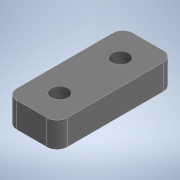
# Autodesk Inventor part: BeltClip
Saved by Autodesk Inventor 2022 (Build 260153000, 153)
## iProperties
Created: 2021-06-25
Part Number: BeltClip
Material: Generic
Document SubType Name: Modeling
Designer: BBL
Density: 1 g/cm^3
Appearance: Gray
Author: BBL
Autodesk Inventor part; units mm, degrees
ref_plane "YZ Plane" through (0, 0, 0) normal (1, 0, 0) x (0, 1, 0)
ref_plane "XZ Plane" through (0, 0, 0) normal (0, 1, 0) x (-1, 0, 0)
ref_plane "XY Plane" through (0, 0, 0) normal (0, 0, 1) x (1, 0, 0)
sketch "Sketch1" plane through (0, 0, 0) normal (0, 1, 0) x (-1, 0, 0)
  circle A0 centre (0, 0) radius 1.65
  circle A1 centre (0, -12) radius 1.65
  line L0 (-5, 5.5) -> (5, 5.5)
  line L1 (5, 5.5) -> (5, -17.5)
  line L2 (5, -17.5) -> (-5, -17.5)
  line L3 (-5, -17.5) -> (-5, 5.5)
  dimension "d0" = 3.3
  dimension "d1" = 3.3
  dimension "d2" = 12
  dimension "d3" = 0
  dimension "d4" = 10
  dimension "d5" = 5
  dimension "d6" = 5.5
  dimension "d7" = 5.5
  constraints: 8 end point, 2 centre point, 2 parallel, 1 coincident, 1 horizontal, 1 perpendicular
  measures "d0" diameter of A0
  measures "d1" diameter of A1
  measures "d2" distance of A1.centre point (0, 0)
  measures "d3" horizontal distance of point (0, 0) A1.centre
  measures "d4" distance of L0.start L0.end
  measures "d5" distance from line of point (0, 0) L3
  measures "d6" distance from line of point (0, 0) L0
  measures "d7" distance from line of L2 A1.centre
extrude "Extrusion1" add sketch "Sketch1" along normal blind 5
fillet "Fillet1" radius 2 4 edges at (5, 2.5, 5.5) (-5, 2.5, 5.5) (5, 2.5, -17.5) (-5, 2.5, -17.5)
body "Solid1"
